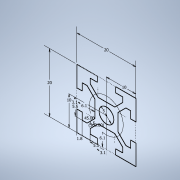
# Autodesk Inventor part: 2020_710
Saved by Autodesk Inventor 2022 (Build 260153000, 153)
## iProperties
Created: 2022-06-12
Part Number: 2020_710
Material: Generic
Document SubType Name: Modeling
Designer: logic
Density: 1 g/cm^3
Appearance: Default
Author: logic
Autodesk Inventor part; units mm, degrees
ref_plane "YZ Plane" through (0, 0, 0) normal (1, 0, 0) x (0, 1, 0)
ref_plane "XZ Plane" through (0, 0, 0) normal (0, 1, 0) x (-1, 0, 0)
ref_plane "XY Plane" through (0, 0, 0) normal (0, 0, 1) x (1, 0, 0)
sketch "Sketch1" plane through (0, 0, 0) normal (0, 0, 1) x (1, 0, 0)
  line L0 (10, -10) -> (-10, -10) construction
  line L1 (-10, -10) -> (-10, 10) construction
  line L2 (-10, 10) -> (10, 10) construction
  line L3 (10, 10) -> (10, -10) construction
  line L4 (-2.8393, -3.9) -> (-5.5, -6.5607)
  line L5 (-5.5, -6.5607) -> (-5.5, -8.2)
  line L6 (-5.5, -8.2) -> (-3.1, -8.2)
  line L7 (-3.1, -8.2) -> (-3.1, -10)
  line L8 (-3.1, -10) -> (-10, -10)
  line L9 (-10, -10) -> (-10, -3.1)
  line L10 (-10, -3.1) -> (-8.2, -3.1)
  line L11 (-8.2, -3.1) -> (-8.2, -5.5)
  line L12 (-8.2, -5.5) -> (-6.5607, -5.5)
  line L13 (-6.5607, -5.5) -> (-3.9, -2.8393)
  line L14 (-2.8393, -3.9) -> (0, -3.9)
  line L15 (-3.9, -2.8393) -> (-3.9, 0)
  line L16 (-3.9, -2.8393) -> (-6.6948, -2.8393) construction
  line L17 (3.9, -2.8393) -> (3.9, 0)
  line L18 (2.8393, -3.9) -> (2.8393, -6.6948) construction
  line L19 (3.9, -2.8393) -> (6.5607, -5.5)
  line L20 (6.5607, -5.5) -> (8.2, -5.5)
  line L21 (5.5, -6.5607) -> (2.8393, -3.9)
  line L22 (5.5, -8.2) -> (5.5, -6.5607)
  line L23 (3.1, -8.2) -> (5.5, -8.2)
  line L24 (3.1, -10) -> (3.1, -8.2)
  line L25 (10, -10) -> (3.1, -10)
  line L26 (10, -3.1) -> (10, -10)
  line L27 (8.2, -3.1) -> (10, -3.1)
  line L28 (8.2, -5.5) -> (8.2, -3.1)
  line L29 (2.8393, -3.9) -> (0, -3.9)
  line L30 (2.8393, 3.9) -> (0, 3.9)
  line L31 (3.9, 2.8393) -> (6.6948, 2.8393) construction
  line L32 (2.8393, 3.9) -> (5.5, 6.5607)
  line L33 (5.5, 6.5607) -> (5.5, 8.2)
  line L34 (6.5607, 5.5) -> (3.9, 2.8393)
  line L35 (8.2, 5.5) -> (6.5607, 5.5)
  line L36 (8.2, 3.1) -> (8.2, 5.5)
  line L37 (10, 3.1) -> (8.2, 3.1)
  line L38 (10, 10) -> (10, 3.1)
  line L39 (3.1, 10) -> (10, 10)
  line L40 (3.1, 8.2) -> (3.1, 10)
  line L41 (5.5, 8.2) -> (3.1, 8.2)
  line L42 (3.9, 2.8393) -> (3.9, 0)
  line L43 (-3.9, 2.8393) -> (-3.9, 0)
  line L44 (-2.8393, 3.9) -> (-2.8393, 6.6948) construction
  line L45 (-3.9, 2.8393) -> (-6.5607, 5.5)
  line L46 (-6.5607, 5.5) -> (-8.2, 5.5)
  line L47 (-5.5, 6.5607) -> (-2.8393, 3.9)
  line L48 (-5.5, 8.2) -> (-5.5, 6.5607)
  line L49 (-3.1, 8.2) -> (-5.5, 8.2)
  line L50 (-3.1, 10) -> (-3.1, 8.2)
  line L51 (-10, 10) -> (-3.1, 10)
  line L52 (-10, 3.1) -> (-10, 10)
  line L53 (-8.2, 3.1) -> (-10, 3.1)
  line L54 (-8.2, 5.5) -> (-8.2, 3.1)
  line L55 (-2.8393, 3.9) -> (0, 3.9)
  circle A0 centre (0, 0) radius 2.5
  point P0 (3.9, 0)
  point P1 (0, 3.9)
  dimension "d0" = 20
  dimension "d1" = 20
  dimension "d2" = 10
  dimension "d3" = 10
  dimension "d4" = 3.1
  dimension "d5" = 5.5
  dimension "d6" = 5.5
  dimension "d7" = 3.1
  dimension "d8" = 1.8
  dimension "d10" = 6.1
  dimension "d11" = 6.1
  dimension "d12" = 45
  dimension "d13" = 1.5
  dimension "d16" = 360
  dimension "d18" = 5
  constraints: 112 end point, 6 perpendicular, 4 horizontal, 3 parallel, 3 vertical, 2 equal length, 1 centre point, 1 coincident, 1 vertical alignment, 109 other
  measures "d0" distance of L1.end L2.end
  measures "d1" distance of L0.end L1.end
  measures "d2" horizontal distance of point (0, 0) L2.end
  measures "d3" horizontal distance of L0.end point (0, 0)
  measures "d4" distance from line of L7 point (0, 0)
  measures "d5" distance from line of L5 point (0, 0)
  measures "d6" distance from line of point (0, 0) L12
  measures "d7" distance from line of point (0, 0) L10
  measures "d8" distance between parallel lines of L1 L11
  measures "d10" distance between parallel lines of L1 L15
  measures "d11" distance between parallel lines of L0 L14
  measures "d12" angle of L16 L13
  measures "d13" distance between parallel lines of L13 L4
  measures "d18" diameter of A0
extrude "Extrusion1" add sketch "Sketch1" along normal blind 710
body "Solid1"
